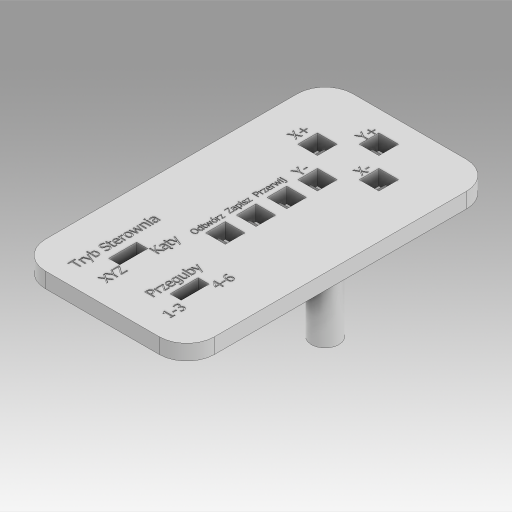
# Autodesk Inventor part: kontroler_top
Saved by Autodesk Inventor 2024.3 (Build 283343000, 343)
## iProperties
Created: 2025-10-11
Part Number: kontroler_top
Material: Ogólny
Document SubType Name: Modeling
Designer: User
Density: 1 g/cm^3
Appearance: Domyślna
Author: User
Autodesk Inventor part; units mm, degrees
(part 1 of 2)
ref_plane "YZ Plane" through (0, 0, 0) normal (1, 0, 0) x (0, 1, 0)
ref_plane "XZ Plane" through (0, 0, 0) normal (0, 1, 0) x (-1, 0, 0)
ref_plane "XY Plane" through (0, 0, 0) normal (0, 0, 1) x (1, 0, 0)
sketch "Szkic1" plane through (0, 0, 0) normal (0, 1, 0) x (-1, 0, 0)
  line L0 (-27.5, 50) -> (27.5, 50)
  line L1 (27.5, 50) -> (27.5, -50)
  line L2 (27.5, -50) -> (-27.5, -50)
  line L3 (-27.5, -50) -> (-27.5, 50)
  line L4 (-27.5, 50) -> (27.5, -50) construction
  line L5 (27.5, 50) -> (-27.5, -50) construction
  line L6 (27.5, 0) -> (-27.5, 0)
  line L7 (-27.5, -50) -> (-27.5, 0)
  circle A0 centre (0, -30) radius 2.5
  line L8 (0, -30) -> (10, -30)
  line L9 (6.8, -26.8) -> (13.2, -26.8)
  line L10 (13.2, -26.8) -> (13.2, -33.2)
  line L11 (13.2, -33.2) -> (6.8, -33.2)
  line L12 (6.8, -33.2) -> (6.8, -26.8)
  line L13 (6.8, -26.8) -> (13.2, -33.2) construction
  line L14 (13.2, -26.8) -> (6.8, -33.2) construction
  line L15 (3.2, -16.8) -> (3.2, -23.2)
  line L16 (-3.2, -16.8) -> (3.2, -16.8)
  line L17 (-3.2, -23.2) -> (-3.2, -16.8)
  line L18 (3.2, -23.2) -> (-3.2, -23.2)
  line L19 (-13.2, -26.8) -> (-6.8, -26.8)
  line L20 (-13.2, -33.2) -> (-13.2, -26.8)
  line L21 (-6.8, -33.2) -> (-13.2, -33.2)
  line L22 (-6.8, -26.8) -> (-6.8, -33.2)
  line L23 (-3.2, -43.2) -> (-3.2, -36.8)
  line L24 (3.2, -43.2) -> (-3.2, -43.2)
  line L25 (3.2, -36.8) -> (3.2, -43.2)
  line L26 (-3.2, -36.8) -> (3.2, -36.8)
  line L27 (-3.2, 3.2) -> (3.2, 3.2)
  line L28 (3.2, 3.2) -> (3.2, -3.2)
  line L29 (3.2, -3.2) -> (-3.2, -3.2)
  line L30 (-3.2, -3.2) -> (-3.2, 3.2)
  line L31 (-3.2, 3.2) -> (3.2, -3.2) construction
  line L32 (3.2, 3.2) -> (-3.2, -3.2) construction
  line L33 (0, 0) -> (0, -10)
  line L34 (-3.2, -6.8) -> (3.2, -6.8)
  line L35 (3.2, -6.8) -> (3.2, -13.2)
  line L36 (3.2, -13.2) -> (-3.2, -13.2)
  line L37 (-3.2, -13.2) -> (-3.2, -6.8)
  line L38 (-3.2, -6.8) -> (3.2, -13.2) construction
  line L39 (3.2, -6.8) -> (-3.2, -13.2) construction
  line L40 (-3.2, 6.8) -> (3.2, 6.8)
  line L41 (3.2, 6.8) -> (3.2, 13.2)
  line L42 (3.2, 13.2) -> (-3.2, 13.2)
  line L43 (-3.2, 13.2) -> (-3.2, 6.8)
  line L44 (0, 13.2) -> (0, 50)
  line L45 (0, 31.6) -> (10, 31.6)
  line L46 (8.2, 36.15) -> (11.8, 36.15)
  line L47 (11.8, 36.15) -> (11.8, 27.05)
  line L48 (11.8, 27.05) -> (8.2, 27.05)
  line L49 (8.2, 27.05) -> (8.2, 36.15)
  line L50 (8.2, 36.15) -> (11.8, 27.05) construction
  line L51 (11.8, 36.15) -> (8.2, 27.05) construction
  line L52 (-8.2, 36.15) -> (-11.8, 36.15)
  line L53 (-11.8, 36.15) -> (-11.8, 27.05)
  line L54 (-11.8, 27.05) -> (-8.2, 27.05)
  line L55 (-8.2, 27.05) -> (-8.2, 36.15)
  dimension "d0" = 55
  dimension "d1" = 100
  dimension "d2" = 5
  dimension "d3" = 10
  dimension "d4" = 6.4
  dimension "d5" = 6.4
  dimension "d8" = 360
  dimension "d10" = 6.4
  dimension "d11" = 6.4
  dimension "d12" = 20
  dimension "d13" = 10
  dimension "d14" = 6.4
  dimension "d15" = 6.4
  dimension "d16" = 10
  dimension "d17" = 3.6
  dimension "d18" = 9.1
  constraints: 112 end point, 15 midpoint, 10 parallel, 8 symmetric about line, 7 horizontal, 5 perpendicular, 1 centre point, 1 collinear, 1 vertical, 33 other
  measures "d0" distance of L1.end L2.end
  measures "d1" distance of L0.end L1.end
  measures "d2" diameter of A0
  measures "d3" distance of L8.start L8.end
  measures "d4" distance of L10.end L11.end
  measures "d5" distance of L9.end L10.end
  measures "d10" distance of L28.end L29.end
  measures "d11" distance of L27.end L28.end
  measures "d12" distance from line of L8.start L2
  measures "d13" distance of L33.start L33.end
  measures "d14" distance of L35.end L36.end
  measures "d15" distance of L34.end L35.end
  measures "d16" distance of L45.start L45.end
  measures "d17" distance of L47.end L48.end
  measures "d18" distance of L46.end L47.end
extrude "Wyciągnięcie proste1" add sketch "Szkic1" along normal blind 5 contours L0 L1 L6 L28 L27 L30 L3 | L6 L30 L29 L28 L1 L2 L3 | A0
sketch "Szkic2" plane through (0, 0, 0) normal (0, -1, 0) x (1, 0, 0)
  point P0 (0, 0)
sketch "Szkic3" plane through (0, 0, 0) normal (0, -1, 0) x (1, 0, 0)
  line L0 (-3.2, 13.2) -> (-3.2, 6.8) projected
  line L1 (-3.2, 10) -> (3.2, 10)
  line L2 (3.2, 6.8) -> (3.2, 13.2) projected
  line L3 (-3.2, 9) -> (3.2, 9)
  line L4 (3.2, 9) -> (3.2, 11)
  line L5 (3.2, 11) -> (-3.2, 11)
  line L6 (-3.2, 11) -> (-3.2, 9)
  line L7 (-3.2, 9) -> (3.2, 11) construction
  line L8 (3.2, 9) -> (-3.2, 11) construction
  line L9 (3.2, 1) -> (-3.2, 1)
  line L10 (-3.2, -1) -> (3.2, -1)
  line L11 (-3.2, 1) -> (-3.2, -1)
  line L12 (3.2, -1) -> (3.2, 1)
  line L13 (3.2, -9) -> (-3.2, -9)
  line L14 (-3.2, -11) -> (3.2, -11)
  line L15 (-3.2, -9) -> (-3.2, -11)
  line L16 (3.2, -11) -> (3.2, -9)
  line L17 (3.2, -19) -> (-3.2, -19)
  line L18 (-3.2, -21) -> (3.2, -21)
  line L19 (-3.2, -19) -> (-3.2, -21)
  line L20 (3.2, -21) -> (3.2, -19)
  circle A0 centre (0, -30) radius 2.5 projected
  circle A1 centre (0, -30) radius 2.5
  line L21 (-9, -33.2) -> (-9, -26.8)
  line L22 (-11, -26.8) -> (-11, -33.2)
  line L23 (-9, -26.8) -> (-11, -26.8)
  line L24 (-11, -33.2) -> (-9, -33.2)
  line L25 (3.2, -39) -> (-3.2, -39)
  line L26 (-3.2, -41) -> (3.2, -41)
  line L27 (-3.2, -39) -> (-3.2, -41)
  line L28 (3.2, -41) -> (3.2, -39)
  line L29 (9, -26.8) -> (9, -33.2)
  line L30 (11, -33.2) -> (11, -26.8)
  line L31 (9, -33.2) -> (11, -33.2)
  line L32 (11, -26.8) -> (9, -26.8)
  line L33 (-11.65, 27.6) -> (-8.35, 27.6)
  line L34 (-8.35, 27.6) -> (-8.35, 35.6)
  line L35 (-8.35, 35.6) -> (-11.65, 35.6)
  line L36 (-11.65, 35.6) -> (-11.65, 27.6)
  line L37 (-11.65, 27.6) -> (-8.35, 35.6) construction
  line L38 (-8.35, 27.6) -> (-11.65, 35.6) construction
  line L39 (3.2, 13.2) -> (-3.2, 13.2) projected
  line L40 (0, 13.2) -> (0, 50)
  line L41 (-27.5, 50) -> (27.5, 50) projected
  line L42 (11.65, 27.6) -> (8.35, 27.6)
  line L43 (8.35, 27.6) -> (8.35, 35.6)
  line L44 (8.35, 35.6) -> (11.65, 35.6)
  line L45 (11.65, 35.6) -> (11.65, 27.6)
  line L46 (11.65, 27.6) -> (8.35, 35.6) construction
  line L47 (8.35, 27.6) -> (11.65, 35.6) construction
  line L48 (-8.2, 27.05) -> (-11.8, 27.05)
  line L49 (-11.8, 27.05) -> (-11.8, 36.15)
  line L50 (-11.8, 36.15) -> (-8.2, 36.15)
  line L51 (-8.2, 36.15) -> (-8.2, 27.05)
  line L52 (-8.2, 27.05) -> (-11.8, 36.15) construction
  line L53 (-11.8, 27.05) -> (-8.2, 36.15) construction
  line L54 (11.65, 27.6) -> (8.35, 27.6)
  line L55 (8.35, 27.6) -> (8.35, 35.6)
  line L56 (8.35, 35.6) -> (11.65, 35.6)
  line L57 (11.65, 35.6) -> (11.65, 27.6)
  line L58 (11.65, 27.6) -> (8.35, 35.6) construction
  line L59 (8.35, 27.6) -> (11.65, 35.6) construction
  line L60 (8.2, 27.05) -> (11.8, 27.05)
  line L61 (11.8, 27.05) -> (11.8, 36.15)
  line L62 (11.8, 36.15) -> (8.2, 36.15)
  line L63 (8.2, 36.15) -> (8.2, 27.05)
  line L64 (8.2, 27.05) -> (11.8, 36.15) construction
  line L65 (11.8, 27.05) -> (8.2, 36.15) construction
  line L66 (27.5, -50) -> (-27.5, -50) projected
  point P0 (0, 0)
  point P1 (0, 10)
  point P2 (-10, 31.6)
  point P3 (10, 31.6)
  dimension "d21" = 6.4
  dimension "d22" = 2
  dimension "d25" = 10
  dimension "d32" = 360
  dimension "d34" = 3.3
  dimension "d35" = 8
  dimension "d38" = 20
  dimension "d39" = 5
  dimension "d40" = 68.416
  dimension "d41" = 85.6
  dimension "d42" = 61
  dimension "d43" = 0
  dimension "d44" = 59
  dimension "d45" = 0
  dimension "d46" = 61
  dimension "d47" = 6.4
  dimension "d48" = 59
  dimension "d49" = 6.4
  constraints: 124 end point, 11 midpoint, 9 symmetric about line, 6 parallel, 3 horizontal, 3 perpendicular, 1 centre point, 1 coincident, 1 vertical, 57 other
  measures "d21" distance of L5.end L4.end
  measures "d22" distance of L4.end L3.end
  measures "d25" distance of L4.end L9.start
  measures "d34" distance of L35.end L34.end
  measures "d35" distance of L34.end L33.end
  measures "d38" distance from line of L66 A0.centre
  measures "d39" diameter of A1
  measures "d40" angle of L66 L64
  measures "d41" distance between parallel lines of L66 L56
  measures "d42" distance from line of point (3.2, 11) L66
  measures "d43" distance from line of point (3.2, 11) L2
  measures "d44" distance from line of point (3.2, 9) L66
  measures "d45" distance from line of point (3.2, 9) L2
  measures "d46" distance from line of point (-3.2, 11) L66
  measures "d47" distance from line of point (-3.2, 11) L2
  measures "d48" distance from line of point (-3.2, 9) L66
  measures "d49" distance from line of point (-3.2, 9) L2
extrude "Wyciągnięcie proste2" add sketch "Szkic3" against normal blind 1.5 contours L5 L2 L1 L0 | L1 L2 L3 L0 | L12 L10 L11 L9 | L16 L14 L15 L13 | L20 L18 L19 L17 | L24 L22 L23 L21 | L28 L26 L27 L25 | L32 L30 L31 L29 | L48 L49 L50 L51 | L63 L62 L61 L60
sketch "Szkic4" plane through (0, 5, 0) normal (0, 1, 0) x (1, 0, 0)
  line L0 (-17.2767, -44.1997) -> (-17.2767, -15.9911) construction
  line L1 (-17.2767, -15.9911) -> (-12.9736, -15.9911) construction
  line L2 (-12.9736, -15.9911) -> (-12.9736, -44.1997) construction
  line L3 (-12.9736, -44.1997) -> (-17.2767, -44.1997) construction
  line L4 (3.3324, -40.0578) -> (3.3324, -22.4746) construction
  line L5 (3.3324, -22.4746) -> (7.9336, -22.4746) construction
  line L6 (7.9336, -22.4746) -> (7.9336, -40.0578) construction
  line L7 (7.9336, -40.0578) -> (3.3324, -40.0578) construction
  line L8 (-8.1301, -43.5227) -> (-8.1301, -36.15) construction
  line L9 (-8.1301, -36.15) -> (-4.1365, -36.15) construction
  line L10 (-4.1365, -36.15) -> (-4.1365, -43.5227) construction
  line L11 (-4.1365, -43.5227) -> (-8.1301, -43.5227) construction
  line L12 (-4.1365, -27.1634) -> (-7.9925, -27.1634) construction
  line L13 (-7.9925, -27.1634) -> (-7.9925, -18.2543) construction
  line L14 (-7.9925, -18.2543) -> (-4.1365, -18.2543) construction
  line L15 (-4.1365, -18.2543) -> (-4.1365, -27.1634) construction
  line L16 (-11.8, -27.05) -> (-8.2, -27.05) projected
  line L17 (-8.2, -27.05) -> (-3.2, -27.05) construction
  line L18 (-8.2, -27.05) -> (-8.2, -36.15) projected
  line L19 (-8.2, -36.15) -> (-3.2, -36.15) construction
  line L20 (16.4473, -43.2657) -> (12.0151, -43.2657) construction
  line L21 (12.0151, -43.2657) -> (12.0151, -36.15) construction
  line L22 (12.0151, -36.15) -> (16.4473, -36.15) construction
  line L23 (16.4473, -36.15) -> (16.4473, -43.2657) construction
  line L24 (16.4473, -27.0005) -> (11.6819, -27.0005) construction
  line L25 (11.6819, -27.0005) -> (11.6819, -19.332) construction
  line L26 (11.6819, -19.332) -> (16.4473, -19.332) construction
  line L27 (16.4473, -19.332) -> (16.4473, -27.0005) construction
  line L28 (-13.8422, 27.6731) -> (-17.7797, 27.6731) construction
  line L29 (-17.7797, 27.6731) -> (-17.7797, 33.1611) construction
  line L30 (-17.7797, 33.1611) -> (-13.8422, 33.1611) construction
  line L31 (-13.8422, 33.1611) -> (-13.8422, 27.6731) construction
  line L32 (6.7627, 28.2297) -> (3.161, 28.2297) construction
  line L33 (3.161, 28.2297) -> (3.161, 33.1611) construction
  line L34 (3.161, 33.1611) -> (6.7627, 33.1611) construction
  line L35 (6.7627, 33.1611) -> (6.7627, 28.2297) construction
  line L36 (-3.2, 18.1022) -> (-6.8497, 18.1022) construction
  line L37 (-6.8497, 18.1022) -> (-6.8497, 22.4735) construction
  line L38 (-6.8497, 22.4735) -> (-3.2, 22.4735) construction
  line L39 (-3.2, 22.4735) -> (-3.2, 18.1022) construction
  line L40 (-2.6732, 38.4003) -> (-6.4043, 38.4003) construction
  line L41 (-6.4043, 38.4003) -> (-6.4043, 43.8486) construction
  line L42 (-6.4043, 43.8486) -> (-2.6732, 43.8486) construction
  line L43 (-2.6732, 43.8486) -> (-2.6732, 38.4003) construction
  line L44 (-3.8579, -3.8627) -> (-6.7158, -3.8627) construction
  line L45 (-6.7158, -3.8627) -> (-6.7158, 4.1729) construction
  line L46 (-6.7158, 4.1729) -> (-3.8579, 4.1729) construction
  line L47 (-3.8579, 4.1729) -> (-3.8579, -3.8627) construction
  line L48 (-3.8579, -15.4827) -> (-6.7165, -15.4827) construction
  line L49 (-6.7165, -15.4827) -> (-6.7165, -5.0858) construction
  line L50 (-6.7165, -5.0858) -> (-3.8579, -5.0858) construction
  line L51 (-3.8579, -5.0858) -> (-3.8579, -15.4827) construction
  line L52 (-3.9582, 5.2833) -> (-6.8168, 5.2833) construction
  line L53 (-6.8168, 5.2833) -> (-6.8168, 15.6802) construction
  line L54 (-6.8168, 15.6802) -> (-3.9582, 15.6802) construction
  line L55 (-3.9582, 15.6802) -> (-3.9582, 5.2833) construction
  spline S0 degree 2 poles (-6.2009, 6.7501) (-6.0713, 6.7501) (-5.8379, 6.6577) (-5.7568, 6.5751) knots 0 0 0 1 2 2 2
  spline S1 degree 2 poles (-5.7568, 6.5751) (-5.6547, 6.4713) (-5.5494, 6.191) (-5.5494, 5.977) knots 0 0 0 1 2 2 2
  line L56 (-5.5494, 5.977) -> (-5.5494, 5.7517)
  line L57 (-5.5494, 5.7517) -> (-4.8038, 5.7517)
  line L58 (-4.8038, 5.7517) -> (-4.8038, 5.4859)
  line L59 (-4.8038, 5.4859) -> (-6.8038, 5.4859)
  line L60 (-6.8038, 5.4859) -> (-6.8038, 5.9884)
  spline S2 degree 2 poles (-6.8038, 5.9884) (-6.8038, 6.1666) (-6.7455, 6.4162) (-6.679, 6.5119) knots 0 0 0 1 2 2 2
  spline S3 degree 2 poles (-6.679, 6.5119) (-6.6029, 6.6237) (-6.3679, 6.7501) (-6.2009, 6.7501) knots 0 0 0 1 2 2 2
  spline S4 degree 2 poles (-6.1928, 6.473) (-6.2965, 6.473) (-6.4489, 6.4017) (-6.4975, 6.3287) knots 0 0 0 1 2 2 2
  spline S5 degree 2 poles (-6.4975, 6.3287) (-6.5397, 6.2655) (-6.5737, 6.097) (-6.5737, 5.9722) knots 0 0 0 1 2 2 2
  line L61 (-6.5737, 5.9722) -> (-6.5737, 5.7517)
  line L62 (-6.5737, 5.7517) -> (-5.7763, 5.7517)
  line L63 (-5.7763, 5.7517) -> (-5.7763, 5.9333)
  spline S6 degree 2 poles (-5.7763, 5.9333) (-5.7763, 6.0953) (-5.8281, 6.2947) (-5.8962, 6.3595) knots 0 0 0 1 2 2 2
  spline S7 degree 2 poles (-5.8962, 6.3595) (-5.9562, 6.4195) (-6.0972, 6.473) (-6.1928, 6.473) knots 0 0 0 1 2 2 2
  line L64 (-6.034, 7.7793) -> (-6.034, 7.7663)
  spline S8 degree 2 poles (-6.034, 7.7663) (-6.0421, 7.7372) (-6.0453, 7.6739) (-6.0453, 7.6302) knots 0 0 0 1 2 2 2
  spline S9 degree 2 poles (-6.0453, 7.6302) (-6.0453, 7.5281) (-5.9562, 7.3271) (-5.8687, 7.2363) knots 0 0 0 1 2 2 2
  line L65 (-5.8687, 7.2363) -> (-4.8038, 7.2363)
  line L66 (-4.8038, 7.2363) -> (-4.8038, 6.9835)
  line L67 (-4.8038, 6.9835) -> (-6.3046, 6.9835)
  line L68 (-6.3046, 6.9835) -> (-6.3046, 7.2363)
  line L69 (-6.3046, 7.2363) -> (-6.081, 7.2363)
  spline S10 degree 2 poles (-6.081, 7.2363) (-6.2042, 7.3741) (-6.3046, 7.5799) (-6.3046, 7.6772) knots 0 0 0 1 2 2 2
  spline S11 degree 2 poles (-6.3046, 7.6772) (-6.3046, 7.7161) (-6.3014, 7.755) (-6.2965, 7.7793) knots 0 0 0 1 2 2 2
  line L70 (-6.2965, 7.7793) -> (-6.034, 7.7793)
  line L71 (-4.8038, 8.9608) -> (-4.8038, 7.8587)
  line L72 (-4.8038, 7.8587) -> (-4.9918, 7.8587)
  line L73 (-4.9918, 7.8587) -> (-6.0972, 8.6431)
  line L74 (-6.0972, 8.6431) -> (-6.0972, 7.8911)
  line L75 (-6.0972, 7.8911) -> (-6.3046, 7.8911)
  line L76 (-6.3046, 7.8911) -> (-6.3046, 8.9462)
  line L77 (-6.3046, 8.9462) -> (-6.1247, 8.9462)
  line L78 (-6.1247, 8.9462) -> (-5.0162, 8.1585)
  line L79 (-5.0162, 8.1585) -> (-5.0162, 8.9608)
  line L80 (-5.0162, 8.9608) -> (-4.8038, 8.9608)
  spline S12 degree 2 poles (-4.7698, 9.849) (-4.7698, 9.4892) (-5.1734, 9.0937) (-5.5461, 9.0937) knots 0 0 0 1 2 2 2
  spline S13 degree 2 poles (-5.5461, 9.0937) (-5.9124, 9.0937) (-6.3468, 9.4778) (-6.3468, 9.7874) knots 0 0 0 1 2 2 2
  spline S14 degree 2 poles (-6.3468, 9.7874) (-6.3468, 9.9268) (-6.2657, 10.1423) (-6.1798, 10.2218) knots 0 0 0 1 2 2 2
  spline S15 degree 2 poles (-6.1798, 10.2218) (-6.0939, 10.3028) (-5.846, 10.3887) (-5.6661, 10.3887) knots 0 0 0 1 2 2 2
  line L81 (-5.6661, 10.3887) -> (-5.5283, 10.3887)
  line L82 (-5.5283, 10.3887) -> (-5.5283, 9.3498)
  spline S16 degree 2 poles (-5.5283, 9.3498) (-5.2674, 9.3498) (-4.9902, 9.6124) (-4.9902, 9.8457) knots 0 0 0 1 2 2 2
  spline S17 degree 2 poles (-4.9902, 9.8457) (-4.9902, 9.9284) (-5.0275, 10.0889) (-5.0567, 10.1537) knots 0 0 0 1 2 2 2
  spline S18 degree 2 poles (-5.0567, 10.1537) (-5.0891, 10.2218) (-5.1458, 10.3158) (-5.1717, 10.3466) knots 0 0 0 1 2 2 2
  line L83 (-5.1717, 10.3466) -> (-5.1717, 10.3611)
  line L84 (-5.1717, 10.3611) -> (-4.8962, 10.3611)
  spline S19 degree 2 poles (-4.8962, 10.3611) (-4.8784, 10.3174) (-4.8265, 10.1845) (-4.8119, 10.1326) knots 0 0 0 1 2 2 2
  spline S20 degree 2 poles (-4.8119, 10.1326) (-4.7909, 10.0597) (-4.7698, 9.9397) (-4.7698, 9.849) knots 0 0 0 1 2 2 2
  spline S21 degree 2 poles (-5.7212, 10.1423) (-5.8233, 10.1391) (-5.9724, 10.097) (-6.0226, 10.0564) knots 0 0 0 1 2 2 2
  spline S22 degree 2 poles (-6.0226, 10.0564) (-6.0794, 10.0127) (-6.1393, 9.8749) (-6.1393, 9.7728) knots 0 0 0 1 2 2 2
  spline S23 degree 2 poles (-6.1393, 9.7728) (-6.1393, 9.6723) (-6.0794, 9.5313) (-6.021, 9.473) knots 0 0 0 1 2 2 2
  spline S24 degree 2 poles (-6.021, 9.473) (-5.961, 9.4162) (-5.8168, 9.3579) (-5.7212, 9.3498) knots 0 0 0 1 2 2 2
  line L85 (-5.7212, 9.3498) -> (-5.7212, 10.1423)
  line L86 (-6.034, 11.4406) -> (-6.034, 11.4276)
  spline S25 degree 2 poles (-6.034, 11.4276) (-6.0421, 11.3984) (-6.0453, 11.3352) (-6.0453, 11.2914) knots 0 0 0 1 2 2 2
  spline S26 degree 2 poles (-6.0453, 11.2914) (-6.0453, 11.1893) (-5.9562, 10.9884) (-5.8687, 10.8976) knots 0 0 0 1 2 2 2
  line L87 (-5.8687, 10.8976) -> (-4.8038, 10.8976)
  line L88 (-4.8038, 10.8976) -> (-4.8038, 10.6448)
  line L89 (-4.8038, 10.6448) -> (-6.3046, 10.6448)
  line L90 (-6.3046, 10.6448) -> (-6.3046, 10.8976)
  line L91 (-6.3046, 10.8976) -> (-6.081, 10.8976)
  spline S27 degree 2 poles (-6.081, 10.8976) (-6.2042, 11.0354) (-6.3046, 11.2412) (-6.3046, 11.3384) knots 0 0 0 1 2 2 2
  spline S28 degree 2 poles (-6.3046, 11.3384) (-6.3046, 11.3773) (-6.3014, 11.4162) (-6.2965, 11.4406) knots 0 0 0 1 2 2 2
  line L92 (-6.2965, 11.4406) -> (-6.034, 11.4406)
  line L93 (-6.3046, 13.4551) -> (-4.8038, 13.0743)
  line L94 (-4.8038, 13.0743) -> (-4.8038, 12.8409)
  line L95 (-4.8038, 12.8409) -> (-5.961, 12.4746)
  line L96 (-5.961, 12.4746) -> (-4.8038, 12.1099)
  line L97 (-4.8038, 12.1099) -> (-4.8038, 11.8782)
  line L98 (-4.8038, 11.8782) -> (-6.3046, 11.494)
  line L99 (-6.3046, 11.494) -> (-6.3046, 11.7566)
  line L100 (-6.3046, 11.7566) -> (-5.1426, 12.0224)
  line L101 (-5.1426, 12.0224) -> (-6.3046, 12.3773)
  line L102 (-6.3046, 12.3773) -> (-6.3046, 12.5864)
  line L103 (-6.3046, 12.5864) -> (-5.1426, 12.9511)
  line L104 (-5.1426, 12.9511) -> (-6.3046, 13.2007)
  line L105 (-6.3046, 13.2007) -> (-6.3046, 13.4551)
  line L106 (-4.8038, 13.9349) -> (-4.8038, 13.682)
  line L107 (-4.8038, 13.682) -> (-6.3046, 13.682)
  line L108 (-6.3046, 13.682) -> (-6.3046, 13.9349)
  line L109 (-6.3046, 13.9349) -> (-4.8038, 13.9349)
  line L110 (-6.5542, 13.9527) -> (-6.5542, 13.6658)
  line L111 (-6.5542, 13.6658) -> (-6.8168, 13.6658)
  line L112 (-6.8168, 13.6658) -> (-6.8168, 13.9527)
  line L113 (-6.8168, 13.9527) -> (-6.5542, 13.9527)
  spline S29 degree 2 poles (-4.7617, 14.7145) (-4.5056, 14.7145) (-4.2366, 14.4389) (-4.2366, 14.1974) knots 0 0 0 1 2 2 2
  spline S30 degree 2 poles (-4.2366, 14.1974) (-4.2366, 14.1553) (-4.2447, 14.0516) (-4.2528, 14.0013) knots 0 0 0 1 2 2 2
  line L114 (-4.2528, 14.0013) -> (-4.4797, 14.0013)
  line L115 (-4.4797, 14.0013) -> (-4.4797, 14.0159)
  spline S31 degree 2 poles (-4.4797, 14.0159) (-4.4732, 14.0451) (-4.4602, 14.1164) (-4.4602, 14.1488) knots 0 0 0 1 2 2 2
  spline S32 degree 2 poles (-4.4602, 14.1488) (-4.4602, 14.2493) (-4.5105, 14.3806) (-4.564, 14.4114) knots 0 0 0 1 2 2 2
  spline S33 degree 2 poles (-4.564, 14.4114) (-4.6126, 14.4422) (-4.7601, 14.4616) (-4.8654, 14.4616) knots 0 0 0 1 2 2 2
  line L116 (-4.8654, 14.4616) -> (-6.0956, 14.4616)
  line L117 (-6.0956, 14.4616) -> (-6.0956, 14.191)
  line L118 (-6.0956, 14.191) -> (-6.3046, 14.191)
  line L119 (-6.3046, 14.191) -> (-6.3046, 14.7145)
  line L120 (-6.3046, 14.7145) -> (-4.7617, 14.7145)
  line L121 (-6.5542, 14.7161) -> (-6.5542, 14.4292)
  line L122 (-6.5542, 14.4292) -> (-6.8168, 14.4292)
  line L123 (-6.8168, 14.4292) -> (-6.8168, 14.7161)
  line L124 (-6.8168, 14.7161) -> (-6.5542, 14.7161)
  spline S34 degree 2 poles (-6.2368, -13.8652) (-6.1039, -13.7517) (-5.7149, -13.6253) (-5.4653, -13.6253) knots 0 0 0 1 2 2 2
  spline S35 degree 2 poles (-5.4653, -13.6253) (-5.2222, -13.6253) (-4.8283, -13.7485) (-4.6954, -13.8652) knots 0 0 0 1 2 2 2
  spline S36 degree 2 poles (-4.6954, -13.8652) (-4.556, -13.9883) (-4.4231, -14.3141) (-4.4231, -14.5102) knots 0 0 0 1 2 2 2
  spline S37 degree 2 poles (-4.4231, -14.5102) (-4.4231, -14.7128) (-4.5609, -15.037) (-4.6954, -15.1553) knots 0 0 0 1 2 2 2
  spline S38 degree 2 poles (-4.6954, -15.1553) (-4.8283, -15.2704) (-5.2189, -15.3935) (-5.4653, -15.3935) knots 0 0 0 1 2 2 2
  spline S39 degree 2 poles (-5.4653, -15.3935) (-5.7165, -15.3935) (-6.099, -15.2687) (-6.2368, -15.1537) knots 0 0 0 1 2 2 2
  spline S40 degree 2 poles (-6.2368, -15.1537) (-6.3697, -15.037) (-6.5074, -14.7112) (-6.5074, -14.5102) knots 0 0 0 1 2 2 2
  spline S41 degree 2 poles (-6.5074, -14.5102) (-6.5074, -14.306) (-6.3648, -13.9786) (-6.2368, -13.8652) knots 0 0 0 1 2 2 2
  spline S42 degree 2 poles (-5.4653, -13.9024) (-5.663, -13.9024) (-5.9693, -13.9883) (-6.0698, -14.0661) knots 0 0 0 1 2 2 2
  spline S43 degree 2 poles (-6.0698, -14.0661) (-6.1736, -14.1456) (-6.2773, -14.3692) (-6.2773, -14.5086) knots 0 0 0 1 2 2 2
  spline S44 degree 2 poles (-6.2773, -14.5086) (-6.2773, -14.6529) (-6.1768, -14.87) (-6.0698, -14.9527) knots 0 0 0 1 2 2 2
  spline S45 degree 2 poles (-6.0698, -14.9527) (-5.9677, -15.0321) (-5.6598, -15.1164) (-5.4653, -15.1164) knots 0 0 0 1 2 2 2
  spline S46 degree 2 poles (-5.4653, -15.1164) (-5.0714, -15.1164) (-4.6533, -14.7858) (-4.6533, -14.5086) knots 0 0 0 1 2 2 2
  spline S47 degree 2 poles (-4.6533, -14.5086) (-4.6533, -14.2315) (-5.0714, -13.9024) (-5.4653, -13.9024) knots 0 0 0 1 2 2 2
  line L125 (-4.4653, -12.199) -> (-4.4653, -12.4519)
  line L126 (-4.4653, -12.4519) -> (-4.6176, -12.4519)
  spline S48 degree 2 poles (-4.6176, -12.4519) (-4.569, -12.5102) (-4.5042, -12.5961) (-4.4766, -12.6545) knots 0 0 0 1 2 2 2
  spline S49 degree 2 poles (-4.4766, -12.6545) (-4.4507, -12.708) (-4.4231, -12.823) (-4.4231, -12.8992) knots 0 0 0 1 2 2 2
  spline S50 degree 2 poles (-4.4231, -12.8992) (-4.4231, -13.0224) (-4.5253, -13.2298) (-4.6241, -13.3028) knots 0 0 0 1 2 2 2
  spline S51 degree 2 poles (-4.6241, -13.3028) (-4.723, -13.3757) (-5.0147, -13.4567) (-5.2043, -13.4567) knots 0 0 0 1 2 2 2
  spline S52 degree 2 poles (-5.2043, -13.4567) (-5.4021, -13.4567) (-5.6906, -13.3546) (-5.7992, -13.2655) knots 0 0 0 1 2 2 2
  spline S53 degree 2 poles (-5.7992, -13.2655) (-5.8964, -13.1828) (-6.0082, -12.9511) (-6.0082, -12.823) knots 0 0 0 1 2 2 2
  spline S54 degree 2 poles (-6.0082, -12.823) (-6.0082, -12.7112) (-5.958, -12.5443) (-5.9061, -12.4519) knots 0 0 0 1 2 2 2
  line L127 (-5.9061, -12.4519) -> (-6.5544, -12.4519)
  line L128 (-6.5544, -12.4519) -> (-6.5544, -12.199)
  line L129 (-6.5544, -12.199) -> (-4.4653, -12.199)
  line L130 (-4.83, -12.4519) -> (-5.6971, -12.4519)
  spline S55 degree 2 poles (-5.6971, -12.4519) (-5.7424, -12.5459) (-5.7765, -12.695) (-5.7765, -12.7809) knots 0 0 0 1 2 2 2
  spline S56 degree 2 poles (-5.7765, -12.7809) (-5.7765, -12.9754) (-5.4847, -13.1958) (-5.2092, -13.1958) knots 0 0 0 1 2 2 2
  spline S57 degree 2 poles (-5.2092, -13.1958) (-4.9434, -13.1958) (-4.663, -13.0272) (-4.663, -12.8409) knots 0 0 0 1 2 2 2
  spline S58 degree 2 poles (-4.663, -12.8409) (-4.663, -12.742) (-4.7538, -12.541) (-4.83, -12.4519) knots 0 0 0 1 2 2 2
  spline S59 degree 2 poles (-4.4361, -11.3789) (-4.4361, -11.5848) (-4.6711, -11.8165) (-4.9256, -11.8165) knots 0 0 0 1 2 2 2
  line L131 (-4.9256, -11.8165) -> (-5.757, -11.8165)
  line L132 (-5.757, -11.8165) -> (-5.757, -11.9867)
  line L133 (-5.757, -11.9867) -> (-5.9661, -11.9867)
  line L134 (-5.9661, -11.9867) -> (-5.9661, -11.8165)
  line L135 (-5.9661, -11.8165) -> (-6.3972, -11.8165)
  line L136 (-6.3972, -11.8165) -> (-6.3972, -11.5637)
  line L137 (-6.3972, -11.5637) -> (-5.9661, -11.5637)
  line L138 (-5.9661, -11.5637) -> (-5.9661, -11.0986)
  line L139 (-5.9661, -11.0986) -> (-5.757, -11.0986)
  line L140 (-5.757, -11.0986) -> (-5.757, -11.5637)
  line L141 (-5.757, -11.5637) -> (-5.0423, -11.5637)
  spline S60 degree 2 poles (-5.0423, -11.5637) (-4.9288, -11.5637) (-4.804, -11.5556) (-4.7505, -11.5281) knots 0 0 0 1 2 2 2
  spline S61 degree 2 poles (-4.7505, -11.5281) (-4.7035, -11.5054) (-4.6565, -11.4033) (-4.6565, -11.3157) knots 0 0 0 1 2 2 2
  spline S62 degree 2 poles (-4.6565, -11.3157) (-4.6565, -11.2541) (-4.6938, -11.1391) (-4.7052, -11.1131) knots 0 0 0 1 2 2 2
  line L142 (-4.7052, -11.1131) -> (-4.7052, -11.0986)
  line L143 (-4.7052, -11.0986) -> (-4.4783, -11.0986)
  spline S63 degree 2 poles (-4.4783, -11.0986) (-4.4588, -11.1699) (-4.4361, -11.3157) (-4.4361, -11.3789) knots 0 0 0 1 2 2 2
  line L144 (-5.9661, -9.0937) -> (-4.4653, -9.4746)
  line L145 (-4.4653, -9.4746) -> (-4.4653, -9.708)
  line L146 (-4.4653, -9.708) -> (-5.6225, -10.0742)
  line L147 (-5.6225, -10.0742) -> (-4.4653, -10.4389)
  line L148 (-4.4653, -10.4389) -> (-4.4653, -10.6707)
  line L149 (-4.4653, -10.6707) -> (-5.9661, -11.0548)
  line L150 (-5.9661, -11.0548) -> (-5.9661, -10.7922)
  line L151 (-5.9661, -10.7922) -> (-4.804, -10.5264)
  line L152 (-4.804, -10.5264) -> (-5.9661, -10.1715)
  line L153 (-5.9661, -10.1715) -> (-5.9661, -9.9624)
  line L154 (-5.9661, -9.9624) -> (-4.804, -9.5977)
  line L155 (-4.804, -9.5977) -> (-5.9661, -9.3482)
  line L156 (-5.9661, -9.3482) -> (-5.9661, -9.0937)
  spline S64 degree 2 poles (-5.2157, -7.6383) (-4.8364, -7.6383) (-4.4231, -8.0029) (-4.4231, -8.3076) knots 0 0 0 1 2 2 2
  spline S65 degree 2 poles (-4.4231, -8.3076) (-4.4231, -8.6204) (-4.8494, -8.9786) (-5.2157, -8.9786) knots 0 0 0 1 2 2 2
  spline S66 degree 2 poles (-5.2157, -8.9786) (-5.5917, -8.9786) (-6.0082, -8.6091) (-6.0082, -8.3076) knots 0 0 0 1 2 2 2
  spline S67 degree 2 poles (-6.0082, -8.3076) (-6.0082, -8.0029) (-5.5933, -7.6383) (-5.2157, -7.6383) knots 0 0 0 1 2 2 2
  spline S68 degree 2 poles (-5.2157, -7.8992) (-5.5074, -7.8992) (-5.7911, -8.1115) (-5.7911, -8.3076) knots 0 0 0 1 2 2 2
  spline S69 degree 2 poles (-5.7911, -8.3076) (-5.7911, -8.5037) (-5.5074, -8.7177) (-5.2157, -8.7177) knots 0 0 0 1 2 2 2
  spline S70 degree 2 poles (-5.2157, -8.7177) (-4.9321, -8.7177) (-4.6403, -8.5037) (-4.6403, -8.3076) knots 0 0 0 1 2 2 2
  spline S71 degree 2 poles (-4.6403, -8.3076) (-4.6403, -8.1131) (-4.9272, -7.8992) (-5.2157, -7.8992) knots 0 0 0 1 2 2 2
  line L157 (-6.7165, -7.8862) -> (-6.2141, -8.2525)
  line L158 (-6.2141, -8.2525) -> (-6.2141, -8.4535)
  line L159 (-6.2141, -8.4535) -> (-6.7165, -8.2136)
  line L160 (-6.7165, -8.2136) -> (-6.7165, -7.8862)
  line L161 (-5.6954, -6.5832) -> (-5.6954, -6.5961)
  spline S72 degree 2 poles (-5.6954, -6.5961) (-5.7035, -6.6253) (-5.7068, -6.6885) (-5.7068, -6.7323) knots 0 0 0 1 2 2 2
  spline S73 degree 2 poles (-5.7068, -6.7323) (-5.7068, -6.8344) (-5.6176, -7.0353) (-5.5301, -7.1261) knots 0 0 0 1 2 2 2
  line L162 (-5.5301, -7.1261) -> (-4.4653, -7.1261)
  line L163 (-4.4653, -7.1261) -> (-4.4653, -7.3789)
  line L164 (-4.4653, -7.3789) -> (-5.9661, -7.3789)
  line L165 (-5.9661, -7.3789) -> (-5.9661, -7.1261)
  line L166 (-5.9661, -7.1261) -> (-5.7424, -7.1261)
  spline S74 degree 2 poles (-5.7424, -7.1261) (-5.8656, -6.9883) (-5.9661, -6.7825) (-5.9661, -6.6853) knots 0 0 0 1 2 2 2
  spline S75 degree 2 poles (-5.9661, -6.6853) (-5.9661, -6.6464) (-5.9629, -6.6075) (-5.958, -6.5832) knots 0 0 0 1 2 2 2
  line L167 (-5.958, -6.5832) -> (-5.6954, -6.5832)
  line L168 (-4.4653, -5.4016) -> (-4.4653, -6.5037)
  line L169 (-4.4653, -6.5037) -> (-4.6533, -6.5037)
  line L170 (-4.6533, -6.5037) -> (-5.7586, -5.7193)
  line L171 (-5.7586, -5.7193) -> (-5.7586, -6.4713)
  line L172 (-5.7586, -6.4713) -> (-5.9661, -6.4713)
  line L173 (-5.9661, -6.4713) -> (-5.9661, -5.4162)
  line L174 (-5.9661, -5.4162) -> (-5.7862, -5.4162)
  line L175 (-5.7862, -5.4162) -> (-4.6776, -6.2039)
  line L176 (-4.6776, -6.2039) -> (-4.6776, -5.4016)
  line L177 (-4.6776, -5.4016) -> (-4.4653, -5.4016)
  line L178 (-4.7028, -2.3846) -> (-4.7028, -3.7817)
  line L179 (-4.7028, -3.7817) -> (-4.9508, -3.7817)
  line L180 (-4.9508, -3.7817) -> (-6.4662, -2.712)
  line L181 (-6.4662, -2.712) -> (-6.4662, -3.7331)
  line L182 (-6.4662, -3.7331) -> (-6.7028, -3.7331)
  line L183 (-6.7028, -3.7331) -> (-6.7028, -2.4121)
  line L184 (-6.7028, -2.4121) -> (-6.463, -2.4121)
  line L185 (-6.463, -2.4121) -> (-4.9395, -3.4932)
  line L186 (-4.9395, -3.4932) -> (-4.9395, -2.3846)
  line L187 (-4.9395, -2.3846) -> (-4.7028, -2.3846)
  spline S76 degree 2 poles (-4.8617, -1.3052) (-4.839, -1.336) (-4.7579, -1.4397) (-4.7336, -1.4883) knots 0 0 0 1 2 2 2
  spline S77 degree 2 poles (-4.7336, -1.4883) (-4.698, -1.5548) (-4.6607, -1.6796) (-4.6607, -1.793) knots 0 0 0 1 2 2 2
  spline S78 degree 2 poles (-4.6607, -1.793) (-4.6607, -1.8854) (-4.7304, -2.0523) (-4.7936, -2.1155) knots 0 0 0 1 2 2 2
  spline S79 degree 2 poles (-4.7936, -2.1155) (-4.8552, -2.1755) (-5.0367, -2.2484) (-5.1372, -2.2484) knots 0 0 0 1 2 2 2
  spline S80 degree 2 poles (-5.1372, -2.2484) (-5.2928, -2.2484) (-5.5132, -2.1172) (-5.5764, -1.9745) knots 0 0 0 1 2 2 2
  spline S81 degree 2 poles (-5.5764, -1.9745) (-5.6348, -1.8481) (-5.6785, -1.5045) (-5.6899, -1.3052) knots 0 0 0 1 2 2 2
  line L188 (-5.6899, -1.3052) -> (-5.7385, -1.3052)
  spline S82 degree 2 poles (-5.7385, -1.3052) (-5.826, -1.3052) (-5.9346, -1.3587) (-5.9654, -1.4073) knots 0 0 0 1 2 2 2
  spline S83 degree 2 poles (-5.9654, -1.4073) (-5.9962, -1.4559) (-6.0156, -1.5953) (-6.0156, -1.6698) knots 0 0 0 1 2 2 2
  spline S84 degree 2 poles (-6.0156, -1.6698) (-6.0156, -1.7574) (-5.9638, -1.994) (-5.9135, -2.1123) knots 0 0 0 1 2 2 2
  line L189 (-5.9135, -2.1123) -> (-5.9135, -2.1269)
  line L190 (-5.9135, -2.1269) -> (-6.1712, -2.1269)
  spline S85 degree 2 poles (-6.1712, -2.1269) (-6.1907, -2.0572) (-6.2393, -1.7963) (-6.2393, -1.6682) knots 0 0 0 1 2 2 2
  spline S86 degree 2 poles (-6.2393, -1.6682) (-6.2393, -1.5126) (-6.1907, -1.3003) (-6.1275, -1.216) knots 0 0 0 1 2 2 2
  spline S87 degree 2 poles (-6.1275, -1.216) (-6.0659, -1.1334) (-5.8698, -1.0523) (-5.7288, -1.0523) knots 0 0 0 1 2 2 2
  line L191 (-5.7288, -1.0523) -> (-4.7028, -1.0523)
  line L192 (-4.7028, -1.0523) -> (-4.7028, -1.3052)
  line L193 (-4.7028, -1.3052) -> (-4.8617, -1.3052)
  line L194 (-5.0724, -1.3052) -> (-5.4889, -1.3052)
  spline S88 degree 2 poles (-5.4889, -1.3052) (-5.4808, -1.3959) (-5.4532, -1.6698) (-5.4273, -1.7557) knots 0 0 0 1 2 2 2
  spline S89 degree 2 poles (-5.4273, -1.7557) (-5.3965, -1.8562) (-5.2685, -1.9875) (-5.155, -1.9875) knots 0 0 0 1 2 2 2
  spline S90 degree 2 poles (-5.155, -1.9875) (-5.0254, -1.9875) (-4.8941, -1.8416) (-4.8941, -1.7023) knots 0 0 0 1 2 2 2
  spline S91 degree 2 poles (-4.8941, -1.7023) (-4.8941, -1.5839) (-4.9962, -1.3895) (-5.0724, -1.3052) knots 0 0 0 1 2 2 2
  spline S92 degree 2 poles (-5.4938, 0.5603) (-5.1178, 0.5603) (-4.6737, 0.2021) (-4.6737, -0.0718) knots 0 0 0 1 2 2 2
  spline S93 degree 2 poles (-4.6737, -0.0718) (-4.6737, -0.1836) (-4.7255, -0.3554) (-4.779, -0.4446) knots 0 0 0 1 2 2 2
  line L195 (-4.779, -0.4446) -> (-4.1502, -0.4446)
  line L196 (-4.1502, -0.4446) -> (-4.1502, -0.6974)
  line L197 (-4.1502, -0.6974) -> (-6.2037, -0.6974)
  line L198 (-6.2037, -0.6974) -> (-6.2037, -0.4446)
  line L199 (-6.2037, -0.4446) -> (-6.0464, -0.4446)
  spline S94 degree 2 poles (-6.0464, -0.4446) (-6.1323, -0.3506) (-6.2458, -0.1204) (-6.2458, 0.0141) knots 0 0 0 1 2 2 2
  spline S95 degree 2 poles (-6.2458, 0.0141) (-6.2458, 0.2718) (-5.8374, 0.5603) (-5.4938, 0.5603) knots 0 0 0 1 2 2 2
  spline S96 degree 2 poles (-5.4646, 0.2994) (-5.7223, 0.2994) (-6.0059, 0.1357) (-6.0059, -0.0475) knots 0 0 0 1 2 2 2
  spline S97 degree 2 poles (-6.0059, -0.0475) (-6.0059, -0.1544) (-5.9103, -0.3554) (-5.8357, -0.4446) knots 0 0 0 1 2 2 2
  line L200 (-5.8357, -0.4446) -> (-4.9832, -0.4446)
  spline S98 degree 2 poles (-4.9832, -0.4446) (-4.9362, -0.3457) (-4.9006, -0.2047) (-4.9006, -0.1139) knots 0 0 0 1 2 2 2
  spline S99 degree 2 poles (-4.9006, -0.1139) (-4.9006, 0.0822) (-5.1891, 0.2994) (-5.4646, 0.2994) knots 0 0 0 1 2 2 2
  line L201 (-4.7028, 1.0806) -> (-4.7028, 0.8277)
  line L202 (-4.7028, 0.8277) -> (-6.2037, 0.8277)
  line L203 (-6.2037, 0.8277) -> (-6.2037, 1.0806)
  line L204 (-6.2037, 1.0806) -> (-4.7028, 1.0806)
  line L205 (-6.4532, 1.0984) -> (-6.4532, 0.8115)
  line L206 (-6.4532, 0.8115) -> (-6.7158, 0.8115)
  line L207 (-6.7158, 0.8115) -> (-6.7158, 1.0984)
  line L208 (-6.7158, 1.0984) -> (-6.4532, 1.0984)
  spline S100 degree 2 poles (-4.6672, 1.8569) (-4.6672, 1.7062) (-4.7482, 1.4452) (-4.7936, 1.3593) knots 0 0 0 1 2 2 2
  line L209 (-4.7936, 1.3593) -> (-5.0772, 1.3593)
  line L210 (-5.0772, 1.3593) -> (-5.0772, 1.3723)
  spline S101 degree 2 poles (-5.0772, 1.3723) (-5.0513, 1.4047) (-4.9897, 1.4922) (-4.9557, 1.5652) knots 0 0 0 1 2 2 2
  spline S102 degree 2 poles (-4.9557, 1.5652) (-4.9249, 1.6284) (-4.8795, 1.784) (-4.8795, 1.8666) knots 0 0 0 1 2 2 2
  spline S103 degree 2 poles (-4.8795, 1.8666) (-4.8795, 1.9266) (-4.9071, 2.0644) (-4.9297, 2.0968) knots 0 0 0 1 2 2 2
  spline S104 degree 2 poles (-4.9297, 2.0968) (-4.9605, 2.1438) (-5.0302, 2.1859) (-5.1015, 2.1859) knots 0 0 0 1 2 2 2
  spline S105 degree 2 poles (-5.1015, 2.1859) (-5.1907, 2.1859) (-5.2831, 2.0887) (-5.3139, 1.9639) knots 0 0 0 1 2 2 2
  spline S106 degree 2 poles (-5.3139, 1.9639) (-5.3252, 1.9152) (-5.3576, 1.7597) (-5.3755, 1.6932) knots 0 0 0 1 2 2 2
  spline S107 degree 2 poles (-5.3755, 1.6932) (-5.4257, 1.5214) (-5.6332, 1.3658) (-5.7806, 1.3658) knots 0 0 0 1 2 2 2
  spline S108 degree 2 poles (-5.7806, 1.3658) (-5.9849, 1.3658) (-6.2393, 1.6721) (-6.2393, 1.925) knots 0 0 0 1 2 2 2
  spline S109 degree 2 poles (-6.2393, 1.925) (-6.2393, 2.0498) (-6.1777, 2.3026) (-6.1307, 2.3885) knots 0 0 0 1 2 2 2
  line L211 (-6.1307, 2.3885) -> (-5.8601, 2.3885)
  line L212 (-5.8601, 2.3885) -> (-5.8601, 2.3755)
  spline S110 degree 2 poles (-5.8601, 2.3755) (-5.9379, 2.2783) (-6.027, 2.0417) (-6.027, 1.9201) knots 0 0 0 1 2 2 2
  spline S111 degree 2 poles (-6.027, 1.9201) (-6.027, 1.7953) (-5.9216, 1.6235) (-5.8163, 1.6235) knots 0 0 0 1 2 2 2
  spline S112 degree 2 poles (-5.8163, 1.6235) (-5.7207, 1.6235) (-5.6283, 1.7256) (-5.5991, 1.8391) knots 0 0 0 1 2 2 2
  spline S113 degree 2 poles (-5.5991, 1.8391) (-5.5845, 1.8942) (-5.5554, 2.0336) (-5.5375, 2.1097) knots 0 0 0 1 2 2 2
  spline S114 degree 2 poles (-5.5375, 2.1097) (-5.4954, 2.2751) (-5.3025, 2.4436) (-5.1356, 2.4436) knots 0 0 0 1 2 2 2
  spline S115 degree 2 poles (-5.1356, 2.4436) (-5.0383, 2.4436) (-4.8665, 2.3674) (-4.8033, 2.2929) knots 0 0 0 1 2 2 2
  spline S116 degree 2 poles (-4.8033, 2.2929) (-4.7369, 2.2135) (-4.6672, 2.0109) (-4.6672, 1.8569) knots 0 0 0 1 2 2 2
  line L213 (-4.7028, 3.664) -> (-4.7028, 2.5619)
  line L214 (-4.7028, 2.5619) -> (-4.8908, 2.5619)
  line L215 (-4.8908, 2.5619) -> (-5.9962, 3.3464)
  line L216 (-5.9962, 3.3464) -> (-5.9962, 2.5943)
  line L217 (-5.9962, 2.5943) -> (-6.2037, 2.5943)
  line L218 (-6.2037, 2.5943) -> (-6.2037, 3.6494)
  line L219 (-6.2037, 3.6494) -> (-6.0237, 3.6494)
  line L220 (-6.0237, 3.6494) -> (-4.9152, 2.8618)
  line L221 (-4.9152, 2.8618) -> (-4.9152, 3.664)
  line L222 (-4.9152, 3.664) -> (-4.7028, 3.664)
  line L223 (-6.4043, 40.8047) -> (-4.7317, 39.7909)
  line L224 (-4.7317, 39.7909) -> (-3.4043, 39.7909)
  line L225 (-3.4043, 39.7909) -> (-3.4043, 39.3922)
  line L226 (-3.4043, 39.3922) -> (-4.6904, 39.3922)
  line L227 (-4.6904, 39.3922) -> (-6.4043, 38.3784)
  line L228 (-6.4043, 38.3784) -> (-6.4043, 38.8209)
  line L229 (-6.4043, 38.8209) -> (-5.0842, 39.594)
  line L230 (-5.0842, 39.594) -> (-6.4043, 40.3817)
  line L231 (-6.4043, 40.3817) -> (-6.4043, 40.8047)
  line L232 (-4.5566, 43.4643) -> (-4.5566, 42.4481)
  line L233 (-4.5566, 42.4481) -> (-3.5404, 42.4481)
  line L234 (-3.5404, 42.4481) -> (-3.5404, 42.1126)
  line L235 (-3.5404, 42.1126) -> (-4.5566, 42.1126)
  line L236 (-4.5566, 42.1126) -> (-4.5566, 41.0964)
  line L237 (-4.5566, 41.0964) -> (-4.88, 41.0964)
  line L238 (-4.88, 41.0964) -> (-4.88, 42.1126)
  line L239 (-4.88, 42.1126) -> (-5.8962, 42.1126)
  line L240 (-5.8962, 42.1126) -> (-5.8962, 42.4481)
  line L241 (-5.8962, 42.4481) -> (-4.88, 42.4481)
  line L242 (-4.88, 42.4481) -> (-4.88, 43.4643)
  line L243 (-4.88, 43.4643) -> (-4.5566, 43.4643)
  line L244 (-6.8497, 20.5066) -> (-5.1771, 19.4928)
  line L245 (-5.1771, 19.4928) -> (-3.8497, 19.4928)
  line L246 (-3.8497, 19.4928) -> (-3.8497, 19.0941)
  line L247 (-3.8497, 19.0941) -> (-5.1358, 19.0941)
  line L248 (-5.1358, 19.0941) -> (-6.8497, 18.0803)
  line L249 (-6.8497, 18.0803) -> (-6.8497, 18.5228)
  line L250 (-6.8497, 18.5228) -> (-5.5296, 19.2959)
  line L251 (-5.5296, 19.2959) -> (-6.8497, 20.0836)
  line L252 (-6.8497, 20.0836) -> (-6.8497, 20.5066)
  line L253 (-4.9802, 21.7975) -> (-4.9802, 20.6622)
  line L254 (-4.9802, 20.6622) -> (-5.3448, 20.6622)
  line L255 (-5.3448, 20.6622) -> (-5.3448, 21.7975)
  line L256 (-5.3448, 21.7975) -> (-4.9802, 21.7975)
  line L257 (6.161, 30.6074) -> (6.161, 30.1503)
  line L258 (6.161, 30.1503) -> (4.9649, 29.421)
  line L259 (4.9649, 29.421) -> (6.161, 28.6771)
  line L260 (6.161, 28.6771) -> (6.161, 28.2468)
  line L261 (6.161, 28.2468) -> (4.6586, 29.2022)
  line L262 (4.6586, 29.2022) -> (3.161, 28.2759)
  line L263 (3.161, 28.2759) -> (3.161, 28.733)
  line L264 (3.161, 28.733) -> (4.3353, 29.4477)
  line L265 (4.3353, 29.4477) -> (3.161, 30.1771)
  line L266 (3.161, 30.1771) -> (3.161, 30.6074)
  line L267 (3.161, 30.6074) -> (4.6392, 29.669)
  line L268 (4.6392, 29.669) -> (6.161, 30.6074)
  line L269 (5.0306, 31.9421) -> (5.0306, 30.8067)
  line L270 (5.0306, 30.8067) -> (4.6659, 30.8067)
  line L271 (4.6659, 30.8067) -> (4.6659, 31.9421)
  line L272 (4.6659, 31.9421) -> (5.0306, 31.9421)
  line L273 (-14.7797, 30.0507) -> (-14.7797, 29.5937)
  line L274 (-14.7797, 29.5937) -> (-15.9758, 28.8643)
  line L275 (-15.9758, 28.8643) -> (-14.7797, 28.1204)
  line L276 (-14.7797, 28.1204) -> (-14.7797, 27.6901)
  line L277 (-14.7797, 27.6901) -> (-16.2821, 28.6455)
  line L278 (-16.2821, 28.6455) -> (-17.7797, 27.7193)
  line L279 (-17.7797, 27.7193) -> (-17.7797, 28.1763)
  line L280 (-17.7797, 28.1763) -> (-16.6055, 28.8911)
  line L281 (-16.6055, 28.8911) -> (-17.7797, 29.6204)
  line L282 (-17.7797, 29.6204) -> (-17.7797, 30.0507)
  line L283 (-17.7797, 30.0507) -> (-16.3016, 29.1123)
  line L284 (-16.3016, 29.1123) -> (-14.7797, 30.0507)
  line L285 (-15.9321, 32.7541) -> (-15.9321, 31.7379)
  line L286 (-15.9321, 31.7379) -> (-14.9158, 31.7379)
  line L287 (-14.9158, 31.7379) -> (-14.9158, 31.4024)
  line L288 (-14.9158, 31.4024) -> (-15.9321, 31.4024)
  line L289 (-15.9321, 31.4024) -> (-15.9321, 30.3862)
  line L290 (-15.9321, 30.3862) -> (-16.2554, 30.3862)
  line L291 (-16.2554, 30.3862) -> (-16.2554, 31.4024)
  line L292 (-16.2554, 31.4024) -> (-17.2716, 31.4024)
  line L293 (-17.2716, 31.4024) -> (-17.2716, 31.7379)
  line L294 (-17.2716, 31.7379) -> (-16.2554, 31.7379)
  line L295 (-16.2554, 31.7379) -> (-16.2554, 32.7541)
  line L296 (-16.2554, 32.7541) -> (-15.9321, 32.7541)
  line L297 (15.0783, -41.3476) -> (15.0783, -42.8111)
  line L298 (15.0783, -42.8111) -> (14.7719, -42.8111)
  line L299 (14.7719, -42.8111) -> (14.7719, -42.2665)
  line L300 (14.7719, -42.2665) -> (12.7614, -42.2665)
  line L301 (12.7614, -42.2665) -> (12.7614, -42.8111)
  line L302 (12.7614, -42.8111) -> (12.4867, -42.8111)
  spline S117 degree 2 poles (12.4867, -42.8111) (12.4867, -42.5023) (12.3117, -42.2106) (12.0685, -42.1912) knots 0 0 0 1 2 2 2
  line L303 (12.0685, -42.1912) -> (12.0685, -41.88)
  line L304 (12.0685, -41.88) -> (14.7719, -41.88)
  line L305 (14.7719, -41.88) -> (14.7719, -41.3476)
  line L306 (14.7719, -41.3476) -> (15.0783, -41.3476)
  line L307 (13.9478, -39.6968) -> (13.9478, -40.8322)
  line L308 (13.9478, -40.8322) -> (13.5831, -40.8322)
  line L309 (13.5831, -40.8322) -> (13.5831, -39.6968)
  line L310 (13.5831, -39.6968) -> (13.9478, -39.6968)
  spline S118 degree 2 poles (12.3627, -38.4886) (12.3627, -38.598) (12.4162, -38.8143) (12.4575, -38.9189) knots 0 0 0 1 2 2 2
  spline S119 degree 2 poles (12.4575, -38.9189) (12.4989, -39.0161) (12.5864, -39.1596) (12.6253, -39.2155) knots 0 0 0 1 2 2 2
  line L311 (12.6253, -39.2155) -> (12.6253, -39.2398)
  line L312 (12.6253, -39.2398) -> (12.1998, -39.2398)
  spline S120 degree 2 poles (12.1998, -39.2398) (12.1293, -39.1085) (12.0151, -38.6587) (12.0151, -38.457) knots 0 0 0 1 2 2 2
  spline S121 degree 2 poles (12.0151, -38.457) (12.0151, -38.2527) (12.0977, -37.9489) (12.1852, -37.8249) knots 0 0 0 1 2 2 2
  spline S122 degree 2 poles (12.1852, -37.8249) (12.2801, -37.6936) (12.5548, -37.5574) (12.7395, -37.5574) knots 0 0 0 1 2 2 2
  spline S123 degree 2 poles (12.7395, -37.5574) (12.9875, -37.5574) (13.3619, -37.8832) (13.4105, -38.1117) knots 0 0 0 1 2 2 2
  line L313 (13.4105, -38.1117) -> (13.4397, -38.1117)
  spline S124 degree 2 poles (13.4397, -38.1117) (13.4591, -38.0169) (13.5467, -37.8006) (13.6342, -37.7082) knots 0 0 0 1 2 2 2
  spline S125 degree 2 poles (13.6342, -37.7082) (13.7193, -37.6158) (13.9916, -37.4991) (14.1885, -37.4991) knots 0 0 0 1 2 2 2
  spline S126 degree 2 poles (14.1885, -37.4991) (14.3903, -37.4991) (14.7331, -37.6377) (14.8643, -37.7641) knots 0 0 0 1 2 2 2
  spline S127 degree 2 poles (14.8643, -37.7641) (15.0005, -37.8954) (15.1415, -38.2673) (15.1415, -38.5031) knots 0 0 0 1 2 2 2
  spline S128 degree 2 poles (15.1415, -38.5031) (15.1415, -38.7292) (15.0321, -39.1717) (14.9567, -39.3224) knots 0 0 0 1 2 2 2
  line L314 (14.9567, -39.3224) -> (14.5313, -39.3224)
  line L315 (14.5313, -39.3224) -> (14.5313, -39.2933)
  spline S129 degree 2 poles (14.5313, -39.2933) (14.6237, -39.1668) (14.7938, -38.739) (14.7938, -38.5275) knots 0 0 0 1 2 2 2
  spline S130 degree 2 poles (14.7938, -38.5275) (14.7938, -38.4035) (14.716, -38.1555) (14.6261, -38.0728) knots 0 0 0 1 2 2 2
  spline S131 degree 2 poles (14.6261, -38.0728) (14.5361, -37.9926) (14.3222, -37.9075) (14.1593, -37.9075) knots 0 0 0 1 2 2 2
  spline S132 degree 2 poles (14.1593, -37.9075) (13.9964, -37.9075) (13.7849, -38.0023) (13.7241, -38.0874) knots 0 0 0 1 2 2 2
  spline S133 degree 2 poles (13.7241, -38.0874) (13.6634, -38.1725) (13.6172, -38.4035) (13.6172, -38.5396) knots 0 0 0 1 2 2 2
  line L316 (13.6172, -38.5396) -> (13.6172, -38.7098)
  line L317 (13.6172, -38.7098) -> (13.2841, -38.7098)
  line L318 (13.2841, -38.7098) -> (13.2841, -38.5761)
  spline S134 degree 2 poles (13.2841, -38.5761) (13.2841, -38.3062) (13.0264, -37.9659) (12.7809, -37.9659) knots 0 0 0 1 2 2 2
  spline S135 degree 2 poles (12.7809, -37.9659) (12.6666, -37.9659) (12.5037, -38.0534) (12.4551, -38.1239) knots 0 0 0 1 2 2 2
  spline S136 degree 2 poles (12.4551, -38.1239) (12.404, -38.1993) (12.3627, -38.384) (12.3627, -38.4886) knots 0 0 0 1 2 2 2
  line L319 (13.7071, -24.8514) -> (13.7071, -25.2088)
  line L320 (13.7071, -25.2088) -> (14.7379, -25.2088)
  line L321 (14.7379, -25.2088) -> (14.7379, -25.5953)
  line L322 (14.7379, -25.5953) -> (13.7071, -25.5953)
  line L323 (13.7071, -25.5953) -> (13.7071, -26.9203)
  line L324 (13.7071, -26.9203) -> (13.284, -26.9203)
  line L325 (13.284, -26.9203) -> (11.7379, -25.5783)
  line L326 (11.7379, -25.5783) -> (11.7379, -25.2088)
  line L327 (11.7379, -25.2088) -> (13.3837, -25.2088)
  line L328 (13.3837, -25.2088) -> (13.3837, -24.8514)
  line L329 (13.3837, -24.8514) -> (13.7071, -24.8514)
  line L330 (13.3837, -25.5953) -> (12.2119, -25.5953)
  line L331 (12.2119, -25.5953) -> (13.3837, -26.6042)
  line L332 (13.3837, -26.6042) -> (13.3837, -25.5953)
  line L333 (13.6074, -23.4316) -> (13.6074, -24.567)
  line L334 (13.6074, -24.567) -> (13.2427, -24.567)
  line L335 (13.2427, -24.567) -> (13.2427, -23.4316)
  line L336 (13.2427, -23.4316) -> (13.6074, -23.4316)
  spline S137 degree 2 poles (13.7654, -21.1367) (13.9964, -21.1367) (14.3878, -21.2898) (14.5191, -21.4187) knots 0 0 0 1 2 2 2
  spline S138 degree 2 poles (14.5191, -21.4187) (14.6576, -21.5524) (14.8011, -21.8879) (14.8011, -22.0896) knots 0 0 0 1 2 2 2
  spline S139 degree 2 poles (14.8011, -22.0896) (14.8011, -22.2914) (14.6649, -22.6245) (14.5288, -22.7509) knots 0 0 0 1 2 2 2
  spline S140 degree 2 poles (14.5288, -22.7509) (14.3659, -22.9065) (13.8189, -23.0815) (13.4202, -23.0815) knots 0 0 0 1 2 2 2
  spline S141 degree 2 poles (13.4202, -23.0815) (13.0288, -23.0815) (12.3991, -22.9211) (12.1657, -22.7533) knots 0 0 0 1 2 2 2
  spline S142 degree 2 poles (12.1657, -22.7533) (11.9372, -22.5905) (11.6819, -22.0751) (11.6819, -21.7371) knots 0 0 0 1 2 2 2
  spline S143 degree 2 poles (11.6819, -21.7371) (11.6819, -21.6375) (11.7014, -21.4624) (11.7233, -21.3968) knots 0 0 0 1 2 2 2
  line L337 (11.7233, -21.3968) -> (12.1098, -21.3968)
  line L338 (12.1098, -21.3968) -> (12.1098, -21.4138)
  spline S144 degree 2 poles (12.1098, -21.4138) (12.0806, -21.4697) (12.0296, -21.6739) (12.0296, -21.7906) knots 0 0 0 1 2 2 2
  spline S145 degree 2 poles (12.0296, -21.7906) (12.0296, -22.165) (12.5353, -22.6245) (13.0312, -22.6683) knots 0 0 0 1 2 2 2
  spline S146 degree 2 poles (13.0312, -22.6683) (12.9315, -22.5248) (12.8221, -22.2234) (12.8221, -22.0435) knots 0 0 0 1 2 2 2
  spline S147 degree 2 poles (12.8221, -22.0435) (12.8221, -21.8684) (12.8926, -21.6059) (12.9996, -21.4624) knots 0 0 0 1 2 2 2
  spline S148 degree 2 poles (12.9996, -21.4624) (13.1236, -21.2971) (13.5077, -21.1367) (13.7654, -21.1367) knots 0 0 0 1 2 2 2
  spline S149 degree 2 poles (13.7824, -21.5451) (13.5977, -21.5451) (13.3473, -21.6423) (13.2597, -21.7493) knots 0 0 0 1 2 2 2
  spline S150 degree 2 poles (13.2597, -21.7493) (13.1965, -21.8295) (13.1552, -22.0289) (13.1552, -22.1334) knots 0 0 0 1 2 2 2
  spline S151 degree 2 poles (13.1552, -22.1334) (13.1552, -22.2744) (13.2403, -22.5394) (13.3205, -22.6683) knots 0 0 0 1 2 2 2
  spline S152 degree 2 poles (13.3205, -22.6683) (13.3643, -22.6707) (13.4469, -22.6755) (13.5101, -22.6755) knots 0 0 0 1 2 2 2
  spline S153 degree 2 poles (13.5101, -22.6755) (13.8213, -22.6755) (14.203, -22.554) (14.3027, -22.4616) knots 0 0 0 1 2 2 2
  spline S154 degree 2 poles (14.3027, -22.4616) (14.3975, -22.3765) (14.4729, -22.1918) (14.4729, -22.0872) knots 0 0 0 1 2 2 2
  spline S155 degree 2 poles (14.4729, -22.0872) (14.4729, -21.8441) (14.1276, -21.5451) (13.7824, -21.5451) knots 0 0 0 1 2 2 2
  line L339 (-4.9925, -24.6715) -> (-4.9925, -25.1893)
  line L340 (-4.9925, -25.1893) -> (-6.388, -26.2858)
  line L341 (-6.388, -26.2858) -> (-6.1911, -26.4608)
  line L342 (-6.1911, -26.4608) -> (-4.9925, -26.4608)
  line L343 (-4.9925, -26.4608) -> (-4.9925, -26.8595)
  line L344 (-4.9925, -26.8595) -> (-7.9925, -26.8595)
  line L345 (-7.9925, -26.8595) -> (-7.9925, -26.4608)
  line L346 (-7.9925, -26.4608) -> (-6.6141, -26.4608)
  line L347 (-6.6141, -26.4608) -> (-7.9925, -25.2307)
  line L348 (-7.9925, -25.2307) -> (-7.9925, -24.7444)
  line L349 (-7.9925, -24.7444) -> (-6.653, -25.9867)
  line L350 (-6.653, -25.9867) -> (-4.9925, -24.6715)
  spline S156 degree 2 poles (-5.2308, -23.208) (-5.1968, -23.2542) (-5.0752, -23.4098) (-5.0387, -23.4827) knots 0 0 0 1 2 2 2
  spline S157 degree 2 poles (-5.0387, -23.4827) (-4.9852, -23.5824) (-4.9293, -23.7696) (-4.9293, -23.9397) knots 0 0 0 1 2 2 2
  spline S158 degree 2 poles (-4.9293, -23.9397) (-4.9293, -24.0783) (-5.0339, -24.3287) (-5.1287, -24.4235) knots 0 0 0 1 2 2 2
  spline S159 degree 2 poles (-5.1287, -24.4235) (-5.2211, -24.5135) (-5.4933, -24.6229) (-5.6441, -24.6229) knots 0 0 0 1 2 2 2
  spline S160 degree 2 poles (-5.6441, -24.6229) (-5.8775, -24.6229) (-6.2081, -24.426) (-6.3029, -24.212) knots 0 0 0 1 2 2 2
  spline S161 degree 2 poles (-6.3029, -24.212) (-6.3904, -24.0224) (-6.4561, -23.507) (-6.4731, -23.208) knots 0 0 0 1 2 2 2
  line L351 (-6.4731, -23.208) -> (-6.546, -23.208)
  spline S162 degree 2 poles (-6.546, -23.208) (-6.6773, -23.208) (-6.8402, -23.2882) (-6.8864, -23.3611) knots 0 0 0 1 2 2 2
  spline S163 degree 2 poles (-6.8864, -23.3611) (-6.9326, -23.4341) (-6.9617, -23.6431) (-6.9617, -23.755) knots 0 0 0 1 2 2 2
  spline S164 degree 2 poles (-6.9617, -23.755) (-6.9617, -23.8863) (-6.8839, -24.2412) (-6.8086, -24.4187) knots 0 0 0 1 2 2 2
  line L352 (-6.8086, -24.4187) -> (-6.8086, -24.4405)
  line L353 (-6.8086, -24.4405) -> (-7.1951, -24.4405)
  spline S165 degree 2 poles (-7.1951, -24.4405) (-7.2243, -24.336) (-7.2972, -23.9446) (-7.2972, -23.7525) knots 0 0 0 1 2 2 2
  spline S166 degree 2 poles (-7.2972, -23.7525) (-7.2972, -23.5192) (-7.2243, -23.2007) (-7.1295, -23.0743) knots 0 0 0 1 2 2 2
  spline S167 degree 2 poles (-7.1295, -23.0743) (-7.0371, -22.9503) (-6.7429, -22.8287) (-6.5314, -22.8287) knots 0 0 0 1 2 2 2
  line L354 (-6.5314, -22.8287) -> (-4.9925, -22.8287)
  line L355 (-4.9925, -22.8287) -> (-4.9925, -23.208)
  line L356 (-4.9925, -23.208) -> (-5.2308, -23.208)
  line L357 (-5.5468, -23.208) -> (-6.1716, -23.208)
  spline S168 degree 2 poles (-6.1716, -23.208) (-6.1595, -23.3441) (-6.1181, -23.755) (-6.0792, -23.8838) knots 0 0 0 1 2 2 2
  spline S169 degree 2 poles (-6.0792, -23.8838) (-6.0331, -24.0346) (-5.841, -24.2315) (-5.6708, -24.2315) knots 0 0 0 1 2 2 2